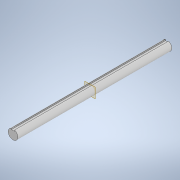
# Autodesk Inventor part: 5x3_8-keyedDriveShaft
Saved by Autodesk Inventor 2021.1 (Build 251245000, 245)
## iProperties
Created: 2020-05-27
Part Number: 5x3_8-keyedDriveShaft
Material: Generic
Document SubType Name: Modeling
Designer: robst
Density: 1 g/cm^3
Appearance: Default
Author: robst
Autodesk Inventor part; units mm, degrees
ref_plane "YZ Plane" through (0, 0, 0) normal (1, 0, 0) x (0, 1, 0)
ref_plane "XZ Plane" through (0, 0, 0) normal (0, 1, 0) x (-1, 0, 0)
sketch "Sketch1" plane through (0, 0, 0) normal (0, 0, 1) x (1, 0, 0)
  arc A0 (-1.5939, 4.4879) -> (1.5939, 4.4879) centre (0, 0) ccw
  line L0 (0, 3.2973) -> (1.5939, 3.2973)
  line L1 (1.5939, 3.2973) -> (1.5939, 4.4879)
  line L2 (0, 4.7625) -> (0, 3.2973) construction
  line L3 (0, 3.2973) -> (-1.5939, 3.2973)
  line L4 (-1.5939, 3.2973) -> (-1.5939, 4.4879)
  dimension "d0" = 9.525
  dimension "d1" = 1.1906
  dimension "d2" = 1.5939
  constraints: 10 end point, 2 point on circle, 2 symmetric about line, 1 centre point, 1 coincident, 1 horizontal, 1 perpendicular, 1 vertical
  measures "d0" diameter of A0
  measures "d1" distance from line of L1.end L0
  measures "d2" distance of L0.end L0.start
extrude "Extrusion1" add sketch "Sketch1" along normal mid plane 152.4
body "Solid1"
